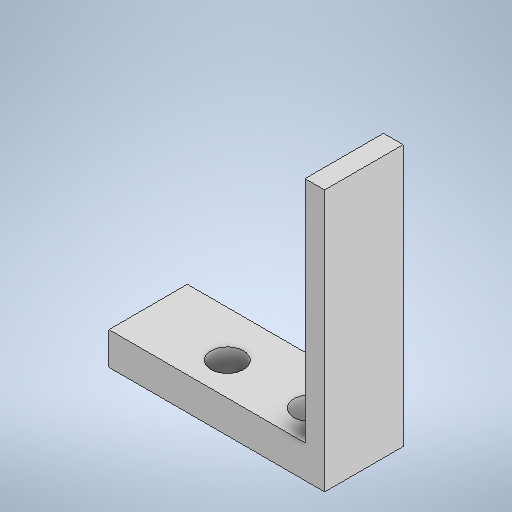
# Autodesk Inventor part: Support
Saved by Autodesk Inventor 2025.1 (Build 291241000, 241)
## iProperties
Created: 2024-11-25
Part Number: Support
Material: Generic
Document SubType Name: Modeling
Designer: hanna
Density: 1 g/cm^3
Appearance: Default
Author: hanna
Autodesk Inventor part; units mm, degrees
ref_plane "YZ Plane" through (0, 0, 0) normal (1, 0, 0) x (0, 1, 0)
ref_plane "XZ Plane" through (0, 0, 0) normal (0, 1, 0) x (-1, 0, 0)
ref_plane "XY Plane" through (0, 0, 0) normal (0, 0, 1) x (1, 0, 0)
sketch "Sketch1" plane through (0, 0, 0) normal (0, 0, 1) x (1, 0, 0)
  line L0 (0, 0) -> (30, 0)
  line L1 (0, 0) -> (0, 5)
  line L2 (0, 5) -> (30, 5)
  line L3 (30, 5) -> (30, 0)
  line L4 (30, 5) -> (30, 40)
  line L5 (30, 40) -> (33, 40)
  line L6 (33, 40) -> (33, 0)
  line L7 (33, 0) -> (30, 0)
  point P0 (23.0555, 5)
  dimension "d0" = 30
  dimension "d2" = 5
  dimension "d11" = 35
  dimension "d12" = 3
  constraints: 16 end point, 3 perpendicular, 3 vertical, 2 horizontal, 1 point on line
  measures "d0" distance of L0.start L0.end
  measures "d2" distance of L0.start L1.end
  measures "d11" distance of L2.end L4.end
  measures "d12" distance of L4.end L5.end
extrude "Extrusion1" add sketch "Sketch1" along normal blind 12
sketch "Sketch2" plane through (0, 0, 0) normal (0, -1, 0) x (1, 0, 0)
  circle A0 centre (25.8, 7) radius 2.125
  line L0 (33, 0) -> (33, 12) projected
  line L1 (0, 12) -> (33, 12) projected
  circle A1 centre (13.1, 7) radius 2.125
  point P0 (0, 0)
  point P1 (33, 6)
  dimension "d13" = 4.25
  dimension "d14" = 7.2
  dimension "d15" = 5
  dimension "d23" = 4.25
  dimension "d24" = 19.9
  dimension "d25" = 5
  constraints: 2 centre point, 1 midpoint
  measures "d13" diameter of A0
  measures "d14" horizontal distance of A0.centre point (33, 6)
  measures "d15" distance from line of L1 A0.centre
  measures "d23" diameter of A1
  measures "d24" distance from line of A1.centre L0
  measures "d25" distance from line of L1 A1.centre
hole "Hole1" at (25.8, 0, 7) at (13.1, 0, 7) direction (0, 1, 0) diameter 5 end through all
body "Solid1"
